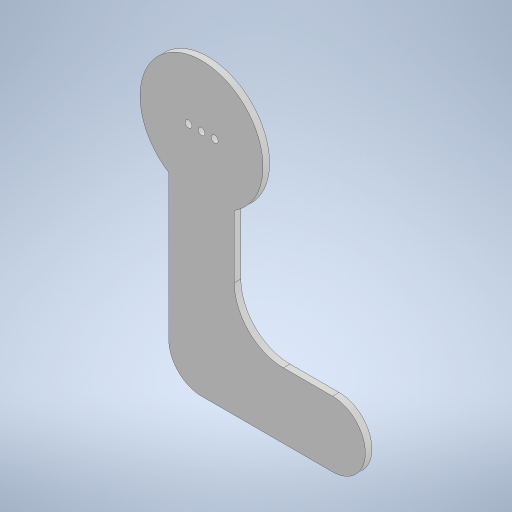
# Autodesk Inventor part: Деталь1
Saved by Autodesk Inventor 2023.1 (Build 271208000, 208)
## iProperties
Created: 2025-10-17
Part Number: Деталь1
Material: Типовые
Document SubType Name: Modeling
Designer: DELL
Density: 1 g/cm^3
Appearance: По умолчанию
Author: DELL
Autodesk Inventor part; units mm, degrees
ref_plane "YZ Plane" through (0, 0, 0) normal (1, 0, 0) x (0, 1, 0)
ref_plane "XZ Plane" through (0, 0, 0) normal (0, 1, 0) x (-1, 0, 0)
ref_plane "XY Plane" through (0, 0, 0) normal (0, 0, 1) x (1, 0, 0)
sketch "Эскиз1" plane through (0, 0, 0) normal (0, 0, 1) x (1, 0, 0)
  circle A0 centre (0, 0) radius 37.5
  circle A1 centre (0, 0) radius 2.1
  circle A2 centre (-8, 0) radius 2.1
  circle A3 centre (8, 0) radius 2.1
  line L0 (0, 0) -> (21.2822, 0) construction
  line L1 (0, 0) -> (-18.9176, 0) construction
  dimension "d0" = 75
  dimension "d1" = 4.2
  dimension "d2" = 4.2
  dimension "d3" = 4.2
  dimension "d4" = 8
  dimension "d5" = 8
  constraints: 4 centre point, 4 end point, 2 coincident, 2 horizontal, 2 point on line
  measures "d0" diameter of A0
  measures "d1" diameter of A1
  measures "d2" diameter of A2
  measures "d3" diameter of A3
  measures "d4" distance of L0.start A3.centre
  measures "d5" distance of L0.start A2.centre
extrude "Выдавливание1" add sketch "Эскиз1" along normal blind 4
sketch "Эскиз2" plane through (0, 0, 4) normal (0, 0, 1) x (1, 0, 0)
  circle A0 centre (0, 0) radius 2.1 construction
  line L0 (0, 0) -> (0, -140) construction
  line L1 (-20, -20) -> (-20, -31.7214) construction
  line L2 (20, -70) -> (20, -31.7214)
  arc A1 (20, -20) -> (-20, -20) centre (0, -20) ccw construction
  arc A2 (-20, -120) -> (0, -140) centre (0, -120) ccw
  line L3 (0, 0) -> (140, 0) construction
  line L4 (0, -120) -> (100, -120) construction
  line L5 (50, -100) -> (80, -100)
  line L6 (80, -140) -> (20, -140)
  arc A3 (80, -140) -> (80, -100) centre (80, -120) ccw
  line L7 (0, -140) -> (20, -140)
  arc A4 (20, -70) -> (50, -100) centre (50, -70) ccw
  arc A5 (37.5, 0) -> (-20, -31.7214) centre (0, 0) ccw construction
  line L8 (-20, -31.7214) -> (-20, -120)
  line L9 (20, -31.7214) -> (20, -20) construction
  arc A6 (20, -31.7214) -> (37.5, 0) centre (0, 0) ccw construction
  arc A7 (-20, -31.7214) -> (20, -31.7214) centre (0, 0) ccw
  point P0 (0, -70)
  point P1 (50, -120)
  dimension "d8" = 140
  dimension "d9" = 90
  dimension "d10" = 40
  dimension "d11" = 100
  dimension "d12" = 40
  dimension "d13" = 30
  constraints: 24 end point, 17 point on circle, 13 tangent, 7 centre point, 5 parallel, 4 point on line, 2 midpoint, 2 perpendicular, 1 coincident, 1 horizontal, 1 vertical
  measures "d8" distance of L0.end L0.start
  measures "d9" angle of L0 L3
  measures "d10" diameter of A2
  measures "d11" distance of L4.start L4.end
  measures "d12" distance between parallel lines of L6 L5
  measures "d13" radius of A4
extrude "Выдавливание2" add sketch "Эскиз2" against normal blind 4
